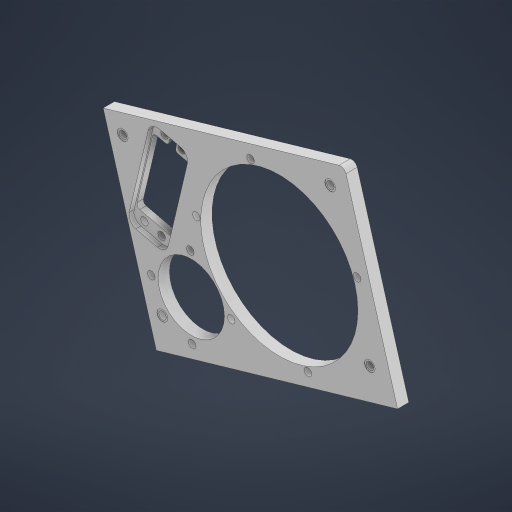
# Autodesk Inventor part: Lower_Plate
Saved by Autodesk Inventor 2024.2 (Build 282272000, 272)
## iProperties
Created: 2024-03-29
Part Number: Lower_Plate
Material: Generic
Document SubType Name: Modeling
Designer: warm
Density: 1 g/cm^3
Appearance: Default
Author: warm
Autodesk Inventor part; units mm, degrees
ref_plane "YZ Plane" through (0, 0, 0) normal (1, 0, 0) x (0, 1, 0)
ref_plane "XZ Plane" through (0, 0, 0) normal (0, 1, 0) x (-1, 0, 0)
ref_plane "XY Plane" through (0, 0, 0) normal (0, 0, 1) x (1, 0, 0)
sketch "Sketch1" plane through (0, 0, 0) normal (0, 0, 1) x (1, 0, 0)
  circle A0 centre (49.935, 18.1273) radius 2.15 projected
  circle A1 centre (22.1322, -42.1716) radius 2.15 projected
  circle A2 centre (-10.364, 45.9302) radius 2.15 projected
  circle A3 centre (-21.2973, -38.0061) radius 2 construction
  circle A4 centre (-43.3867, -61.1591) radius 2 construction
  circle A5 centre (-66.5396, -39.0697) radius 2 construction
  circle A6 centre (-44.4503, -15.9167) radius 2 construction
  circle A7 centre (-21.2973, -38.0061) radius 2.15
  circle A8 centre (-43.3867, -61.1591) radius 2.15
  circle A9 centre (-66.5396, -39.0697) radius 2.15
  circle A10 centre (-44.4503, -15.9167) radius 2.15
  line L0 (72.7593, -34.944) -> (-63.7175, -74.4952)
  circle A11 centre (22.1322, -42.1716) radius 7.15 construction
  circle A12 centre (-43.3867, -61.1591) radius 7.15 construction
  circle A13 centre (49.935, 18.1273) radius 7.15 construction
  circle A14 centre (-10.364, 45.9302) radius 7.15 construction
  line L1 (72.7593, -34.944) -> (42.7074, 68.7545)
  line L2 (61.4193, 4.1865) -> (59.0868, 12.2348)
  line L3 (42.7074, 68.7545) -> (-93.7695, 29.2033)
  circle A15 centre (-66.5396, -39.0697) radius 7.15 construction
  line L4 (-63.7175, -74.4952) -> (-93.7695, 29.2033)
  arc A16 (26.2989, -37.6054) -> (49.1681, 11.9935) centre (5.8841, 1.8793) ccw construction
  circle A17 centre (5.8841, 1.8793) radius 44.45
  arc A18 (-43.4778, -57.2827) -> (-49.2361, -56.518) centre (-43.9185, -38.5379) ccw construction
  circle A19 centre (-43.9185, -38.5379) radius 18.75
  circle A20 centre (-41.0626, 2.5767) radius 2.15 projected
  point P0 (0, 0)
  dimension "d4" = 4.3
  dimension "d5" = 4.3
  dimension "d6" = 4.3
  dimension "d7" = 4.3
  dimension "d8" = 5
  dimension "d10" = 0
  dimension "d11" = 5
  dimension "d12" = 5
  dimension "d13" = 0
  dimension "d14" = 5
  dimension "d15" = 5
  constraints: 10 end point, 9 centre point, 9 coincident, 5 tangent, 4 point on line, 2 parallel, 1 perpendicular, 6 other
  measures "d4" diameter of A7
  measures "d5" diameter of A8
  measures "d6" diameter of A9
  measures "d7" diameter of A10
  measures "d8" radial gap between concentric circles of A1 A11
  measures "d10" distance of A4.centre A12.centre
  measures "d11" radial gap between concentric circles of A8 A12
  measures "d12" radial gap between concentric circles of A13 A0
  measures "d13" distance of A2.centre A14.centre
  measures "d14" radial gap between concentric circles of A14 A2
  measures "d15" radial gap between concentric circles of A15 A9
extrude "Extrusion1" add sketch "Sketch1" against normal blind 6.35
sketch "Sketch3" plane through (0, 0, 0) normal (0, 0, 1) x (1, 0, 0)
  line L0 (-61.3029, 24.5377) -> (-55.2691, 23.1116)
  line L1 (-55.2691, 23.1116) -> (-55.1667, 23.5451)
  arc A0 (-55.1667, 23.5451) -> (-61.2004, 24.9712) centre (-59.9421, 16.8177) ccw
  line L2 (-61.2004, 24.9712) -> (-61.3029, 24.5377)
  arc A1 (-66.2644, 27.4572) -> (-68.0692, 26.3425) centre (-66.6094, 25.9974) ccw
  line L3 (-66.2644, 27.4572) -> (-49.5256, 23.501)
  arc A2 (-48.4108, 21.6962) -> (-49.5256, 23.501) centre (-49.8706, 22.0412) ccw
  line L4 (-48.4108, 21.6962) -> (-57.1054, -15.0903)
  arc A3 (-58.9102, -16.2051) -> (-57.1054, -15.0903) centre (-58.5652, -14.7453) ccw
  line L5 (-58.9102, -16.2051) -> (-75.649, -12.2488)
  arc A4 (-76.7638, -10.444) -> (-75.649, -12.2488) centre (-75.304, -10.789) ccw
  line L6 (-76.7638, -10.444) -> (-68.0692, 26.3425)
  line L7 (-48.0658, 23.1559) -> (-67.7242, 27.8022)
  line L8 (-67.7242, 27.8022) -> (-66.1486, 34.4686)
  line L9 (-66.1486, 34.4686) -> (-46.4902, 29.8223)
  line L10 (-46.4902, 29.8223) -> (-48.0658, 23.1559)
  line L11 (-48.0658, 23.1559) -> (-48.4722, 21.4367)
  line L12 (-67.7242, 27.8022) -> (-68.3933, 24.9712)
  line L13 (-52.7581, 3.3029) -> (-72.4165, 7.9492) construction
  line L14 (-75.649, -12.2488) -> (-58.9102, -16.2051)
  line L15 (-57.4504, -16.5501) -> (-77.1088, -11.9038)
  line L16 (-77.1088, -11.9038) -> (-78.6844, -18.5701)
  line L17 (-78.6844, -18.5701) -> (-59.026, -23.2164)
  line L18 (-59.026, -23.2164) -> (-57.4504, -16.5501)
  line L19 (-57.4504, -16.5501) -> (-57.1054, -15.0903)
  line L20 (-77.1088, -11.9038) -> (-76.7638, -10.444)
  line L21 (-59.026, -23.2164) -> (-78.6844, -18.5701)
  line L22 (-78.6844, -18.5701) -> (-66.1486, 34.4686)
  line L23 (-66.1486, 34.4686) -> (-46.4902, 29.8223)
  line L24 (-46.4902, 29.8223) -> (-59.026, -23.2164)
  line L25 (-56.9137, -19.8007) -> (-46.1306, 25.8223)
  line L26 (-49.9059, 31.9346) -> (-62.1486, 34.8282)
  line L27 (-68.2609, 31.0529) -> (-79.044, -14.5701)
  line L28 (-75.2687, -20.6824) -> (-63.026, -23.576)
  arc A5 (-46.1306, 25.8223) -> (-49.9059, 31.9346) centre (-51.0744, 26.9908) ccw
  arc A6 (-62.1486, 34.8282) -> (-68.2609, 31.0529) centre (-63.3171, 29.8844) ccw
  arc A7 (-63.026, -23.576) -> (-56.9137, -19.8007) centre (-61.8575, -18.6322) ccw
  arc A8 (-79.044, -14.5701) -> (-75.2687, -20.6824) centre (-74.1002, -15.7386) ccw
  point P0 (0, 0)
  point P1 (-58.0822, -24.7445)
  point P2 (-44.9621, 30.7661)
  point P3 (-67.0924, 35.9966)
  point P4 (-80.2125, -19.5139)
  point P5 (-66.2644, 27.4572)
  point P6 (-46.5937, 29.3844)
  point P7 (-46.928, 29.9257)
  point P8 (-65.7107, 34.3651)
  point P9 (-66.2521, 34.0307)
  point P10 (-78.5809, -18.1323)
  point P11 (-78.2466, -18.6736)
  point P12 (-59.4639, -23.1129)
  point P13 (-58.9226, -22.7786)
  dimension "d18" = 6.85
  dimension "d19" = 0
  dimension "d20" = 0
  dimension "d23" = 1.27
  dimension "d24" = 1.27
  dimension "d25" = 9.62
  dimension "d26" = 21.47
  dimension "d27" = 8.12
  dimension "d28" = 5.08
  constraints: 58 end point, 18 point on circle, 10 point on line, 9 centre point, 8 tangent, 6 parallel, 4 symmetric about line, 3 equal radius, 2 midpoint, 2 perpendicular, 1 collinear, 29 other
  measures "d18" distance of L7.end L8.end
  measures "d19" distance between parallel lines of L4 L10
  measures "d20" distance between parallel lines of L6 L8
  measures "d23" distance between parallel lines of L24 L25
  measures "d24" distance between parallel lines of L17 L28
  measures "d25" distance from line of A4.centre L28
  measures "d26" distance between parallel lines of L18 L27
  measures "d27" distance between parallel lines of L26 L3
  measures "d28" radius of A5
extrude "Extrusion2" cut sketch "Sketch3" against normal blind 2.725 contours L2 A0 L1 L0 | L3 A2 L4 A3 L5 A4 L6 A1 | L7 L8 A6 L9 A5 L10 L3 | A1 L12 L7 | L6 L20 L16 A8 L27 A6 L8 L12 | L7 L11 A2 | L11 L10 A5 L25 A7 L18 L19 L4 | A4 L15 L20 | A6 L26 A5 L9 | L5 L15 L18 A7 L17 A8 L16 | L19 L15 A3 | L17 A7 L28 A8
sketch "Sketch4" plane through (0, 0, -2.725) normal (0, 0, 1) x (1, 0, 0)
  line L0 (-61.3029, 24.5377) -> (-55.2691, 23.1116) construction
  line L1 (-55.2691, 23.1116) -> (-55.1667, 23.5451) construction
  arc A0 (-55.1667, 23.5451) -> (-61.2004, 24.9712) centre (-59.9421, 16.8177) ccw construction
  line L2 (-61.2004, 24.9712) -> (-61.3029, 24.5377) construction
  line L3 (-66.2644, 27.4572) -> (-49.5256, 23.501)
  arc A1 (-48.4108, 21.6962) -> (-49.5256, 23.501) centre (-49.8706, 22.0412) ccw construction
  line L4 (-46.9502, 27.8759) -> (-48.4108, 21.6962) construction
  arc A2 (-46.9502, 27.8759) -> (-48.4366, 30.2823) centre (-48.8966, 28.3359) ccw construction
  line L5 (-49.9937, 30.6503) -> (-48.4366, 30.2823) construction
  line L6 (-50.1677, 29.9142) -> (-49.9937, 30.6503) construction
  arc A3 (-53.0872, 30.6042) -> (-50.1677, 29.9142) centre (-52.0285, 28.5624) ccw construction
  line L7 (-52.9132, 31.3404) -> (-53.0872, 30.6042) construction
  line L8 (-59.7255, 32.9505) -> (-52.9132, 31.3404) construction
  line L9 (-59.8995, 32.2143) -> (-59.7255, 32.9505) construction
  arc A4 (-62.8191, 32.9044) -> (-59.8995, 32.2143) centre (-61.7604, 30.8625) ccw construction
  line L10 (-62.6451, 33.6405) -> (-62.8191, 32.9044) construction
  line L11 (-64.2022, 34.0085) -> (-62.6451, 33.6405) construction
  arc A5 (-64.2022, 34.0085) -> (-66.6086, 32.5222) centre (-64.6622, 32.0622) ccw construction
  line L12 (-68.0692, 26.3425) -> (-66.6086, 32.5222) construction
  arc A6 (-66.2644, 27.4572) -> (-68.0692, 26.3425) centre (-66.6094, 25.9974) ccw construction
  line L13 (-48.4108, 21.6962) -> (-57.1054, -15.0903) construction
  arc A7 (-60.9724, -22.7564) -> (-58.566, -21.2701) centre (-60.5124, -20.81) ccw construction
  line L14 (-60.9724, -22.7564) -> (-62.5295, -22.3884) construction
  line L15 (-62.5295, -22.3884) -> (-62.3555, -21.6522) construction
  arc A8 (-62.3555, -21.6522) -> (-65.2751, -20.9622) centre (-63.4143, -19.6104) ccw construction
  line L16 (-65.2751, -20.9622) -> (-65.4491, -21.6983) construction
  line L17 (-65.4491, -21.6983) -> (-72.2614, -20.0882) construction
  line L18 (-72.2614, -20.0882) -> (-72.0874, -19.3521) construction
  arc A9 (-72.0874, -19.3521) -> (-75.007, -18.662) centre (-73.1461, -17.3102) ccw construction
  line L19 (-75.007, -18.662) -> (-75.181, -19.3982) construction
  line L20 (-75.181, -19.3982) -> (-76.738, -19.0301) construction
  arc A10 (-78.2244, -16.6237) -> (-76.738, -19.0301) centre (-76.278, -17.0838) ccw construction
  line L21 (-78.2244, -16.6237) -> (-76.7638, -10.444) construction
  line L22 (-76.7638, -10.444) -> (-68.0692, 26.3425) construction
  arc A11 (-58.9102, -16.2051) -> (-57.1054, -15.0903) centre (-58.5652, -14.7453) ccw construction
  line L23 (-58.9102, -16.2051) -> (-75.649, -12.2488) construction
  arc A12 (-76.7638, -10.444) -> (-75.649, -12.2488) centre (-75.304, -10.789) ccw construction
  circle A13 centre (-52.0285, 28.5624) radius 2.15
  circle A14 centre (-61.7604, 30.8625) radius 2.15
  circle A15 centre (-63.4143, -19.6104) radius 2.15
  circle A16 centre (-73.1461, -17.3102) radius 2.15
  line L24 (-54.4118, 21.5218) -> (-54.1473, 22.641) construction
  line L25 (-62.5167, 24.6191) -> (-62.7812, 23.4999) construction
  circle A17 centre (-52.0285, 28.5624) radius 3 construction
  circle A18 centre (-61.7604, 30.8625) radius 3 construction
  line L26 (-55.9486, 25.0191) -> (-59.8414, 25.9391) construction
  line L27 (-59.8414, 25.9391) -> (-58.5579, 31.3695)
  line L28 (-58.5579, 31.3695) -> (-54.6651, 30.4494)
  line L29 (-54.6651, 30.4494) -> (-55.9486, 25.0191)
  line L30 (-56.4874, -15.2364) -> (-47.7929, 21.5501)
  arc A19 (-47.7929, 21.5501) -> (-49.3795, 24.1189) centre (-49.8706, 22.0412) ccw
  line L31 (-49.3795, 24.1189) -> (-66.1183, 28.0752)
  arc A20 (-66.1183, 28.0752) -> (-68.6872, 26.4885) centre (-66.6094, 25.9974) ccw
  line L32 (-68.6872, 26.4885) -> (-77.3818, -10.2979)
  line L33 (-77.3818, -10.2979) -> (-78.8424, -16.4777)
  arc A21 (-78.8424, -16.4777) -> (-76.8841, -19.6481) centre (-76.278, -17.0838) ccw
  line L34 (-76.8841, -19.6481) -> (-74.709, -20.1622)
  line L35 (-74.709, -20.1622) -> (-74.3152, -18.4958)
  arc A22 (-72.6316, -18.8937) -> (-74.3152, -18.4958) centre (-73.1461, -17.3102) ccw
  line L36 (-72.6316, -18.8937) -> (-73.0254, -20.5601)
  line L37 (-73.0254, -20.5601) -> (-64.9772, -22.4624)
  line L38 (-64.9772, -22.4624) -> (-64.5833, -20.7959)
  arc A23 (-62.8997, -21.1939) -> (-64.5833, -20.7959) centre (-63.4143, -19.6104) ccw
  line L39 (-62.8997, -21.1939) -> (-63.2936, -22.8603)
  line L40 (-63.2936, -22.8603) -> (-61.1185, -23.3744)
  arc A24 (-61.1185, -23.3744) -> (-57.948, -21.4161) centre (-60.5124, -20.81) ccw
  line L41 (-75.7951, -12.8668) -> (-59.0563, -16.823)
  arc A25 (-59.0563, -16.823) -> (-56.4874, -15.2364) centre (-58.5652, -14.7453) ccw
  line L42 (-56.4874, -15.2364) -> (-47.7929, 21.5501)
  line L43 (-47.7929, 21.5501) -> (-46.3323, 27.7298)
  arc A26 (-46.3323, 27.7298) -> (-48.2905, 30.9003) centre (-48.8966, 28.3359) ccw
  line L44 (-48.2905, 30.9003) -> (-50.4656, 31.4144)
  line L45 (-50.4656, 31.4144) -> (-50.8594, 29.7479)
  arc A27 (-52.5431, 30.1459) -> (-50.8594, 29.7479) centre (-52.0285, 28.5624) ccw
  line L46 (-52.5431, 30.1459) -> (-52.1492, 31.8123)
  line L47 (-52.1492, 31.8123) -> (-60.1975, 33.7145)
  line L48 (-60.1975, 33.7145) -> (-60.5913, 32.0481)
  arc A28 (-62.2749, 32.446) -> (-60.5913, 32.0481) centre (-61.7604, 30.8625) ccw
  line L49 (-62.2749, 32.446) -> (-61.8811, 34.1124)
  line L50 (-61.8811, 34.1124) -> (-64.0561, 34.6265)
  arc A29 (-64.0561, 34.6265) -> (-67.2266, 32.6683) centre (-64.6622, 32.0622) ccw
  line L51 (-67.2266, 32.6683) -> (-68.6872, 26.4885)
  line L52 (-68.6872, 26.4885) -> (-77.3818, -10.2979)
  arc A30 (-77.3818, -10.2979) -> (-75.7951, -12.8668) centre (-75.304, -10.789) ccw
  point P0 (0, 0)
  point P1 (-56.3194, 32.1454)
  point P2 (-55.8026, 25.637)
  point P3 (-59.6953, 26.5571)
  point P4 (-74.4407, -19.0268)
  point P5 (-72.7571, -19.4247)
  point P6 (-64.7088, -21.327)
  point P7 (-63.0252, -21.7249)
  point P8 (-77.3818, -10.2979)
  dimension "d29" = 4.3
  dimension "d30" = 4.3
  dimension "d31" = 4.3
  dimension "d32" = 4.3
  dimension "d33" = 6
  dimension "d34" = 6
  dimension "d35" = 1.27
  dimension "d36" = 0
  dimension "d39" = 0.635
  dimension "d41" = 0.635
  constraints: 102 end point, 50 point on circle, 31 centre point, 6 coincident, 2 parallel, 2 tangent, 1 collinear, 1 midpoint, 1 perpendicular, 119 other
  measures "d29" diameter of A13
  measures "d30" diameter of A14
  measures "d31" diameter of A15
  measures "d32" diameter of A16
  measures "d33" diameter of A17
  measures "d34" diameter of A18
  measures "d35" distance from line of point (-56.319, 32.145) L28
  measures "d36" distance between parallel lines of L3 L26
  measures "d39" distance between parallel lines of L13 L30
  measures "d41" distance between parallel lines of L23 L41
extrude "Extrusion3" cut sketch "Sketch4" against normal through all contours L27 L31 L29 L3 | L3 L29 L31 A19 L30 A25 L41 A30 L32 A20 L27 | L27 L28 L29 L31 | A15 L39 A23 L38 | L38 A23 L39 A15 | A16 L36 A22 L35 | L35 A22 L36 A16 | L49 A28 L48 A14 | A14 L48 A28 L49 | L45 A27 L46 A13 | A13 L46 A27 L45
fillet "Fillet1" radius 1.5875 4 edges at (-55.8026, 25.637, -4.5375) (-54.6651, 30.4494, -4.5375) (-58.5579, 31.3695, -4.5375) (-59.6953, 26.5571, -4.5375)
fillet "Fillet2" radius 3.175 1 edges at (42.7074, 68.7545, -3.175)
sketch "Sketch5" plane through (0, 0, 0) normal (0, 0, 1) x (1, 0, 0)
  circle A0 centre (57.0512, -21.713) radius 2.15 projected
  circle A1 centre (34.6484, 55.5908) radius 2.15 projected
  circle A2 centre (-82.7345, 21.5731) radius 2.15 projected
  circle A3 centre (-60.3318, -55.7307) radius 2.15 projected
  circle A4 centre (57.0512, -21.713) radius 3.05
  circle A5 centre (34.6484, 55.5908) radius 3.05
  circle A6 centre (-82.7345, 21.5731) radius 3.05
  circle A7 centre (-60.3318, -55.7307) radius 3.05
  point P0 (0, 0)
  dimension "d43" = 6.1
  dimension "d44" = 6.1
  dimension "d45" = 6.1
  dimension "d46" = 6.1
  constraints: 4 centre point, 4 coincident
  measures "d43" diameter of A4
  measures "d44" diameter of A5
  measures "d45" diameter of A6
  measures "d46" diameter of A7
extrude "Extrusion4" cut sketch "Sketch5" against normal blind 0.15
sketch "Sketch6" plane through (-60.3318, -55.7307, 0) normal (0, 0, 1) x (1, 0, 0)
  circle A0 centre (-22.4027, 77.3038) radius 2.15 projected
  circle A1 centre (94.9802, 111.3215) radius 2.15 projected
  circle A2 centre (117.383, 34.0177) radius 2.15 projected
  circle A3 centre (0, 0) radius 2.15 projected
  point P0 (60.3318, 55.7307)
extrude "Extrusion5" cut sketch "Sketch6" against normal through all
body "Solid1"
